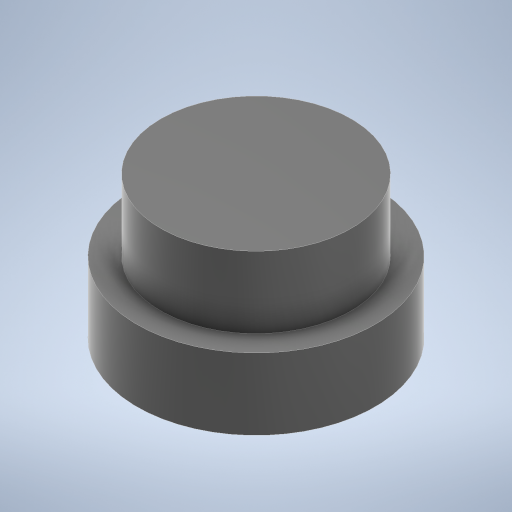
# Autodesk Inventor part: Speaker
Saved by Autodesk Inventor 2023 (Build 270158000, 158)
## iProperties
Created: 2022-11-17
Part Number: Speaker
Material: Generic
Document SubType Name: Modeling
Designer: spfow
Density: 1 g/cm^3
Appearance: Smooth - Black
Author: spfow
Autodesk Inventor part; units mm, degrees
ref_plane "YZ Plane" through (0, 0, 0) normal (1, 0, 0) x (0, 1, 0)
ref_plane "XZ Plane" through (0, 0, 0) normal (0, 1, 0) x (-1, 0, 0)
ref_plane "XY Plane" through (0, 0, 0) normal (0, 0, 1) x (1, 0, 0)
sketch "Sketch1" plane through (0, 0, 0) normal (0, 1, 0) x (-1, 0, 0)
  circle A0 centre (0, 0) radius 5.08
  circle A1 centre (0, 0) radius 6.35
  dimension "d0" = 10.16
  dimension "d1" = 12.7
  constraints: 2 centre point, 2 coincident
  measures "d0" diameter of A0
  measures "d1" diameter of A1
extrude "Extrusion1" add sketch "Sketch1" along normal blind 7.62 contours A0
extrude "Extrusion2" add sketch "Sketch1" along normal blind 3.81
body "Solid1"
